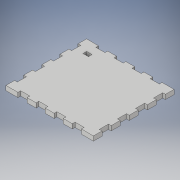
# Autodesk Inventor part: BackPlateBase
Saved by Autodesk Inventor 2019.4 (Build 234330000, 330)
## iProperties
Created: 2020-06-30
Part Number: BackPlateBase
Material: Generic
Document SubType Name: Modeling
Designer: wimva
Density: 1 g/cm^3
Appearance: Default
Author: wimva
Autodesk Inventor part; units mm, degrees
ref_plane "YZ Plane" through (0, 0, 0) normal (1, 0, 0) x (0, 1, 0)
ref_plane "XZ Plane" through (0, 0, 0) normal (0, 1, 0) x (-1, 0, 0)
ref_plane "XY Plane" through (0, 0, 0) normal (0, 0, 1) x (1, 0, 0)
sketch "Sketch2" plane through (0, 0, 0) normal (0, 1, 0) x (-1, 0, 0)
  line L0 (-48.26, 44.5) -> (48.26, 44.5)
  line L1 (48.26, 44.5) -> (48.26, -44.5)
  line L2 (48.26, -44.5) -> (-48.26, -44.5)
  line L3 (-48.26, -44.5) -> (-48.26, 44.5)
  line L4 (-48.26, 44.5) -> (48.26, -44.5) construction
  line L5 (48.26, 44.5) -> (-48.26, -44.5) construction
  point P0 (0, 0)
  dimension "d0" = 96.52
  dimension "d1" = 89
  constraints: 12 end point, 2 midpoint, 2 parallel, 1 horizontal, 1 perpendicular
  measures "d0" distance of L1.end L2.end
  measures "d1" distance of L0.end L1.end
extrude "Extrusion1" add sketch "Sketch2" along normal blind 5
sketch "Sketch3" plane through (0, 5, 0) normal (0, 1, 0) x (1, 0, 0)
  line L0 (48.26, 44.5) -> (-48.26, 44.5) construction
  line L1 (-15, 44.5) -> (-5, 44.5)
  line L2 (-5, 44.5) -> (-5, 41.5)
  line L3 (-5, 41.5) -> (-15, 41.5)
  line L4 (-15, 41.5) -> (-15, 44.5)
  line L5 (0, 62.3) -> (0, -62.3) construction
  point P0 (0, 0)
  dimension "d4" = 10
  dimension "d5" = 3
  dimension "d6" = 5
  constraints: 8 end point, 2 parallel, 1 horizontal, 1 perpendicular, 1 point on line
  measures "d4" distance of L2.end L3.end
  measures "d5" distance of L1.end L2.end
  measures "d6" distance between parallel lines of L5 L2
extrude "Extrusion2" cut sketch "Sketch3" against normal through all
pattern_linear "Rectangular Pattern1" count 2 spacing 20 along (-1, 0, 0) count 2 spacing 40 along (1, 0, 0) of "Extrusion2"
mirror "Mirror1" about plane through (0, 0, 0) normal (0, 0, 1) of "Extrusion2", "Rectangular Pattern1"
sketch "Sketch4" plane through (0, 5, 0) normal (0, 1, 0) x (1, 0, 0)
  line L0 (-48.26, 44.5) -> (-48.26, -44.5) construction
  line L1 (-48.26, 5) -> (-45.26, 5)
  line L2 (-45.26, 5) -> (-45.26, 15)
  line L3 (-45.26, 15) -> (-48.26, 15)
  line L4 (-48.26, 15) -> (-48.26, 5)
  line L5 (67.564, 0) -> (-67.564, 0) construction
  point P0 (0, 0)
  dimension "d15" = 3
  dimension "d16" = 10
  dimension "d17" = 5
  constraints: 8 end point, 2 parallel, 1 horizontal, 1 perpendicular, 1 point on line
  measures "d15" distance of L3.end L2.end
  measures "d16" distance of L1.end L2.end
  measures "d17" distance between parallel lines of L5 L1
extrude "Extrusion3" cut sketch "Sketch4" against normal through all
pattern_linear "Rectangular Pattern2" count 2 spacing 20 along (0, 0, -1) count 2 spacing 40 along (0, 0, 1) of "Extrusion3"
mirror "Mirror2" about plane through (0, 0, 0) normal (1, 0, 0) of "Extrusion3", "Rectangular Pattern2"
sketch "Sketch5" plane through (0, 5, 0) normal (0, 1, 0) x (1, 0, 0)
  line L0 (-36.26, 32.5) -> (-30.26, 32.5)
  line L1 (-30.26, 32.5) -> (-30.26, 28.5)
  line L2 (-30.26, 28.5) -> (-36.26, 28.5)
  line L3 (-36.26, 28.5) -> (-36.26, 32.5)
  line L4 (-35, 44.5) -> (-48.26, 44.5) construction
  line L5 (-48.26, 25) -> (-48.26, 15) construction
  point P0 (0, 0)
  dimension "d26" = 6
  dimension "d27" = 4
  dimension "d28" = 12
  dimension "d29" = 12
  constraints: 8 end point, 2 parallel, 1 horizontal, 1 perpendicular
  measures "d26" distance of L1.end L2.end
  measures "d27" distance of L0.end L1.end
  measures "d28" distance between parallel lines of L0 L4
  measures "d29" distance between parallel lines of L3 L5
extrude "Extrusion4" cut sketch "Sketch5" against normal through all
equation "\"d0\" = ModuleWidth"
equation "\"d1\" = ModuleHeight"
equation "\"d2\" = ModuleBottomThickness"
equation "\"d4\" = ModuleCaseSlotWidth"
equation "\"d5\" = ModuleCaseSlotDepth"
equation "\"d6\" = 0.5 * ModuleCaseSlotWidth"
equation "\"d7\" = ModuleBottomThickness"
equation "\"d11\" = 2 * ModuleCaseSlotWidth"
equation "\"d14\" = 4 * ModuleCaseSlotWidth"
equation "\"d15\" = ModuleCaseSlotDepth"
equation "\"d16\" = ModuleCaseSlotWidth"
equation "\"d17\" = 0.5 * ModuleCaseSlotWidth"
equation "\"d18\" = ModuleBottomThickness"
equation "\"d22\" = 2 * ModuleCaseSlotWidth"
equation "\"d25\" = 4 * ModuleCaseSlotWidth"
equation "\"d26\" = ModuleConnectorWidth"
equation "\"d27\" = ModuleConnectorDepth"
equation "\"d30\" = ModuleBottomThickness"
equation "\"RackWidth\" = 482.6"
equation "\"U\" = 44.5"
equation "\"ModuleWidth\" = 96.52"
equation "\"ModuleHeight\" = 89"
equation "\"ModuleCaseThickness\" = 3"
equation "\"ModuleBottomThickness\" = 5"
equation "\"ModuleCaseSlotDepth\" = 3"
equation "\"ModuleCaseSlotWidth\" = 10"
equation "\"LaserThickness\" = 0"
equation "\"ModuleConnectorHeight\" = 6"
equation "\"ModuleConnectorWidth\" = 6"
equation "\"ModuleConnectorDepth\" = 4"
equation "\"ModuleConnectorHoleWidth\" = 6"
equation "\"ModuleConnectorHoleHeight\" = 4"
body "Solid1"
